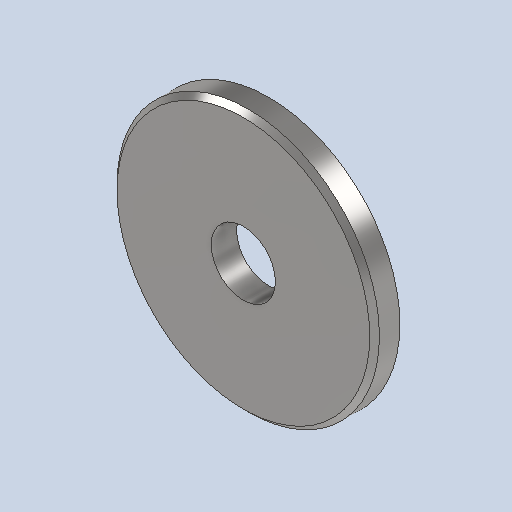
# Autodesk Inventor part: Flansch_Wellennabeverbindung_Klemmdeckel
Saved by Autodesk Inventor 2024 (Build 280153000, 153)
## iProperties
Created: 2022-07-14
Part Number: Flansch_Wellennabeverbindung_Klemmdeckel
Material: Edelstahl
Document SubType Name: Modeling
Designer: alexw
Density: 8 g/cm^3
Appearance: Halbpoliert
Mass: 11.1138 g
Surface Area: 13.2597 cm^2
Volume: 1.38922 cm^3
Author: alexw
Autodesk Inventor part; units mm, degrees
ref_plane "YZ Plane" through (0, 0, 0) normal (1, 0, 0) x (0, 1, 0)
ref_plane "XZ Plane" through (0, 0, 0) normal (0, 1, 0) x (-1, 0, 0)
ref_plane "XY Plane" through (0, 0, 0) normal (0, 0, 1) x (1, 0, 0)
sketch "Skizze1" plane through (0, 0, 0) normal (0, 0, 1) x (1, 0, 0)
  circle A0 centre (0, 0) radius 13.5
  dimension "d0" = 27
  constraints: 1 centre point, 1 coincident
  measures "d0" diameter of A0
extrude "Extrusion1" add sketch "Skizze1" along normal blind 2.6
chamfer "Fase1" distance 0.5 angle 45 1 edges at (-13.5, 0, 2.6)
sketch "Skizze2" plane through (0, 0, 0) normal (0, 0, -1) x (-1, 0, 0)
  point P0 (0, 0)
  point P1 (0, 0)
  constraints: 1 coincident
hole "Bohrung1" at (0, 0, 0) direction (0, 0, 1) diameter 6.6 depth 30 tip angle 118 clearance for "Flachkopfsenkschraube DIN EN ISO 2009" size "M6" standard "DIN"
equation "\"d0\" = Flansch_Klemmdeckelausnahme_Dia"
equation "\"KlemmdeckelHeight\" = 3"
equation "\"Flansch_Klemmdeckelausnahme_Dia\" = 27"
